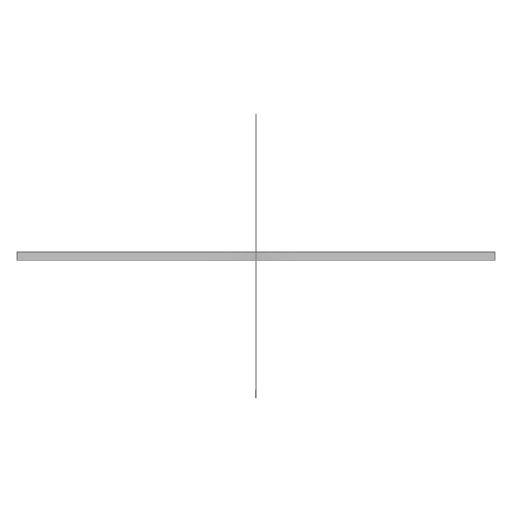
# Autodesk Inventor part: PLETINA DE INERCIA
Saved by Autodesk Inventor 2024 (Build 280153000, 153)
## iProperties
Created: 2024-06-13
Part Number: PLETINA DE INERCIA
Material: Generic
Document SubType Name: Modeling
Designer: Jhuliams
Density: 1 g/cm^3
Appearance: Default
Author: Jhuliams
Autodesk Inventor part; units mm, degrees
ref_plane "YZ Plane" through (0, 0, 0) normal (1, 0, 0) x (0, 1, 0)
ref_plane "XZ Plane" through (0, 0, 0) normal (0, 1, 0) x (-1, 0, 0)
ref_plane "XY Plane" through (0, 0, 0) normal (0, 0, 1) x (1, 0, 0)
sketch "Sketch2" plane through (0, 0, 0) normal (0, 1, 0) x (-1, 0, 0)
  line L0 (0, 0) -> (419.3143, 419.3143)
  line L1 (0, 0) -> (593, 0) construction
  line L2 (0, 0) -> (-419.3143, -419.3143)
  line L3 (419.3143, 419.3143) -> (-419.3143, 419.3143)
  line L4 (-419.3143, 419.3143) -> (-419.3143, -419.3143)
  line L5 (-419.3143, -419.3143) -> (419.3143, -419.3143)
  line L6 (419.3143, -419.3143) -> (419.3143, 419.3143)
  line L7 (419.3143, -419.3143) -> (-419.3143, 419.3143)
  line L8 (418.4304, -420.1982) -> (-420.1982, 418.4304)
  line L9 (420.1982, -418.4304) -> (-418.4304, 420.1982)
  line L10 (420.1982, 418.4304) -> (0.8839, -0.8839)
  line L11 (0.8839, -0.8839) -> (-418.4304, -420.1982)
  line L12 (418.4304, 420.1982) -> (-0.8839, 0.8839)
  line L13 (-0.8839, 0.8839) -> (-420.1982, -418.4304)
  point P0 (0, 1.7678)
  point P1 (-417.5466, 419.3143)
  point P2 (-419.3143, 417.5466)
  point P3 (-1.7678, 0)
  point P4 (-417.5466, -419.3143)
  point P5 (0, -1.7678)
  point P6 (-419.3143, -417.5466)
  point P7 (1.7678, 0)
  point P8 (419.3143, 417.5466)
  point P9 (417.5466, 419.3143)
  point P10 (417.5466, -419.3143)
  point P11 (419.3143, -417.5466)
  dimension "d4" = 593
  dimension "d5" = 45
  dimension "d6" = 593
  dimension "d7" = 1.25
  dimension "d8" = 1.25
  dimension "d9" = 1.25
  dimension "d10" = 1.25
  constraints: 28 end point, 4 parallel, 2 horizontal, 1 equal length, 1 perpendicular, 2 other
  measures "d4" distance of L0.start L0.end
  measures "d5" angle of L1 L0
  measures "d6" distance of L0.start L2.end
  measures "d7" distance between parallel lines of L7 L8
  measures "d8" distance between parallel lines of L7 L9
  measures "d9" distance between parallel lines of L0 L10
  measures "d10" distance between parallel lines of L0 L12
extrude "Extrusion2" add sketch "Sketch2" along normal blind 25 contours L9 L12 L3 L0 | L0 L6 L10 L9 | L8 L11 L5 L2 | L2 L4 L13 L8 | L10 L9 L6 L7 | L7 L5 L8 L11 | L13 L8 L4 L7 | L7 L3 L9 L12
body "Solid2"
